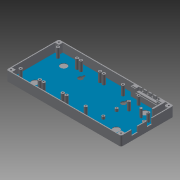
# Autodesk Inventor part: bottom-case
Saved by Autodesk Inventor 2015 (Build 190159000, 159)
## iProperties
Created: 2016-04-25
Part Number: bottom-case
Material: 一般
Document SubType Name: Modeling
Designer: yamashita1
Density: 1 g/cm^3
Appearance: 既定
Author: yamashita1
Autodesk Inventor part; units mm, degrees
ref_plane "YZ Plane" through (0, 0, 0) normal (1, 0, 0) x (0, 1, 0)
ref_plane "XZ Plane" through (0, 0, 0) normal (0, 1, 0) x (-1, 0, 0)
ref_plane "XY Plane" through (0, 0, 0) normal (0, 0, 1) x (1, 0, 0)
sketch "スケッチ1" plane through (0, 0, 0) normal (0, 0, 1) x (1, 0, 0)
  line L0 (-120, 55) -> (120, 55)
  line L1 (120, 55) -> (120, -55)
  line L2 (120, -55) -> (-120, -55)
  line L3 (-120, -55) -> (-120, 55)
  point P0 (0, 0)
  dimension "d0" = 240
  dimension "d1" = 110
  dimension "d2" = 120
  dimension "d3" = 55
  constraints: 8 end point, 2 parallel, 1 horizontal, 1 perpendicular
  measures "d0" distance of L1.end L2.end
  measures "d1" distance of L0.end L1.end
  measures "d2" distance from line of L3 point (0, 0)
  measures "d3" distance from line of L2 point (0, 0)
extrude "押し出し1" add sketch "スケッチ1" along normal blind 20
sketch "スケッチ2" plane through (0, 0, 20) normal (0, 0, 1) x (1, 0, 0)
  line L0 (-118, 53) -> (118, 53)
  line L1 (118, 53) -> (118, -53)
  line L2 (118, -53) -> (-118, -53)
  line L3 (-118, -53) -> (-118, 53)
  point P0 (0, 0)
  dimension "d6" = 236
  dimension "d7" = 106
  dimension "d8" = 118
  dimension "d9" = 53
  constraints: 8 end point, 2 parallel, 1 horizontal, 1 perpendicular
  measures "d6" distance of L1.end L2.end
  measures "d7" distance of L0.end L1.end
  measures "d8" distance from line of L3 point (0, 0)
  measures "d9" distance from line of L2 point (0, 0)
extrude "押し出し2" cut sketch "スケッチ2" against normal blind 18
sketch "スケッチ3" plane through (0, 0, 2) normal (0, 0, 1) x (1, 0, 0)
  line L0 (-118, 53) -> (-110, 53)
  line L1 (-110, 53) -> (-110, 45)
  line L2 (-110, 45) -> (-118, 45)
  line L3 (-118, 45) -> (-118, 53)
  line L4 (-118, -53) -> (-110, -53)
  line L5 (-110, -53) -> (-110, -45)
  line L6 (-110, -45) -> (-118, -45)
  line L7 (-118, -45) -> (-118, -53)
  line L8 (118, -53) -> (110, -53)
  line L9 (110, -53) -> (110, -45)
  line L10 (110, -45) -> (118, -45)
  line L11 (118, -45) -> (118, -53)
  line L12 (118, 53) -> (110, 53)
  line L13 (110, 53) -> (110, 45)
  line L14 (110, 45) -> (118, 45)
  line L15 (118, 45) -> (118, 53)
  point P0 (0, 0)
  dimension "d13" = 8
  dimension "d14" = 8
  dimension "d15" = 8
  dimension "d16" = 8
  dimension "d17" = 8
  dimension "d18" = 8
  dimension "d19" = 8
  dimension "d117" = 8
  constraints: 32 end point, 8 parallel, 4 horizontal, 4 perpendicular
  measures "d13" distance of L0.end L1.end
  measures "d14" distance of L6.end L5.end
  measures "d15" distance of L5.end L4.end
  measures "d16" distance of L9.end L10.end
  measures "d17" distance of L8.end L9.end
  measures "d18" distance of L14.end L13.end
  measures "d19" distance of L13.end L12.end
  measures "d117" distance from line of L3 L1.end
extrude "押し出し3" add sketch "スケッチ3" along normal blind 18
sketch "スケッチ4" plane through (0, 0, 20) normal (0, 0, 1) x (1, 0, 0)
  circle A0 centre (-115, 50) radius 1.6
  line L0 (-120, 55) -> (-120, -55) projected
  line L1 (120, 55) -> (-120, 55) projected
  circle A1 centre (-115, -50) radius 1.6
  line L2 (-120, -55) -> (120, -55) projected
  circle A2 centre (115, 50) radius 1.6
  line L3 (120, -55) -> (120, 55) projected
  circle A3 centre (115, -50) radius 1.6
  point P0 (0, 0)
  dimension "d22" = 3.2
  dimension "d23" = 5
  dimension "d24" = 5
  dimension "d25" = 3.2
  dimension "d26" = 5
  dimension "d27" = 5
  dimension "d28" = 3.2
  dimension "d29" = 5
  dimension "d30" = 5
  dimension "d31" = 3.2
  dimension "d32" = 5
  dimension "d33" = 5
  constraints: 4 centre point
  measures "d22" diameter of A0
  measures "d23" distance from line of L0 A0.centre
  measures "d24" distance from line of L1 A0.centre
  measures "d25" diameter of A1
  measures "d26" distance from line of L0 A1.centre
  measures "d27" distance from line of L2 A1.centre
  measures "d28" diameter of A2
  measures "d29" distance from line of L1 A2.centre
  measures "d30" distance from line of L3 A2.centre
  measures "d31" diameter of A3
  measures "d32" distance from line of L3 A3.centre
  measures "d33" distance from line of L2 A3.centre
extrude "押し出し4" cut sketch "スケッチ4" against normal blind 20 contours A0 | A1 | A2 | A3
sketch "スケッチ5" plane through (0, 0, 0) normal (0, 0, -1) x (-1, 0, 0)
  circle A0 centre (115, -50) radius 3.5
  circle A1 centre (115, -50) radius 1.6 projected
  circle A2 centre (115, 50) radius 3.5
  circle A3 centre (115, 50) radius 1.6 projected
  circle A4 centre (-115, 50) radius 3.5
  circle A5 centre (-115, 50) radius 1.6 projected
  circle A6 centre (-115, -50) radius 3.5
  circle A7 centre (-115, -50) radius 1.6 projected
  point P0 (0, 0)
  dimension "d36" = 7
  dimension "d37" = 7
  dimension "d38" = 7
  dimension "d39" = 7
  constraints: 4 centre point, 4 concentric
  measures "d36" diameter of A0
  measures "d37" diameter of A2
  measures "d38" diameter of A4
  measures "d39" diameter of A6
extrude "押し出し5" cut sketch "スケッチ5" against normal blind 15
sketch "スケッチ6" plane through (0, 0, 2) normal (0, 0, 1) x (1, 0, 0)
  circle A0 centre (-10, -39) radius 3.25
  circle A1 centre (-10, 39) radius 3.25
  circle A2 centre (30, 39) radius 3.25
  circle A3 centre (30, -39) radius 3.25
  point P0 (0, 0)
  dimension "d42" = 39
  dimension "d43" = 10
  dimension "d44" = 40
  dimension "d45" = 39
  dimension "d46" = 6.5
  dimension "d47" = 6.5
  dimension "d48" = 6.5
  dimension "d49" = 6.5
  constraints: 4 centre point, 4 coincident, 2 horizontal alignment, 2 vertical alignment
  measures "d42" vertical distance of point (-10, -39) point (0, 0)
  measures "d43" horizontal distance of point (-10, -39) point (0, 0)
  measures "d44" distance of point (30, -39) point (-10, -39)
  measures "d45" vertical distance of point (-10, 39) point (0, 0)
  measures "d46" diameter of A0
  measures "d47" diameter of A1
  measures "d48" diameter of A2
  measures "d49" diameter of A3
extrude "押し出し6" add sketch "スケッチ6" along normal blind 19.4
sketch "スケッチ7" plane through (-10, 39, 21.4) normal (0, 0, 1) x (1, 0, 0)
  circle A0 centre (0, 0) radius 1.4
  circle A1 centre (0, 0) radius 3.25 projected
  circle A2 centre (0, -78) radius 1.4
  circle A3 centre (0, -78) radius 3.25 projected
  circle A4 centre (40, 0) radius 1.4
  circle A5 centre (40, 0) radius 3.25 projected
  circle A6 centre (40, -78) radius 1.4
  circle A7 centre (40, -78) radius 3.25 projected
  point P0 (10, -39)
  dimension "d52" = 2.8
  dimension "d53" = 2.8
  dimension "d54" = 2.8
  dimension "d55" = 2.8
  constraints: 4 centre point, 4 concentric
  measures "d52" diameter of A0
  measures "d53" diameter of A2
  measures "d54" diameter of A4
  measures "d55" diameter of A6
extrude "押し出し7" cut sketch "スケッチ7" against normal blind 10 contours A0 | A2 | A4 | A6
pattern_linear "矩形状パターン1" count 3 spacing 48 along (-1, 0, 0) of "押し出し6", "押し出し7"
sketch "スケッチ8" plane through (120, -55, 0) normal (1, 0, 0) x (0, 0, -1)
  line L0 (-20, 100) -> (-20, 10) projected
  line L1 (-20, 21.9) -> (-9, 21.9)
  line L2 (-9, 21.9) -> (-9, 34.9)
  line L3 (-9, 34.9) -> (-20, 34.9)
  line L4 (-20, 34.9) -> (-20, 21.9)
  line L5 (-20, 0) -> (-20, 110) projected
  line L6 (-20, 54.515) -> (-9, 54.515)
  line L7 (-9, 54.515) -> (-9, 64.515)
  line L8 (-9, 64.515) -> (-20, 64.515)
  line L9 (-20, 64.515) -> (-20, 54.515)
  point P0 (0, 55)
  point P1 (-20, 66.5)
  point P2 (-20, 59.515)
  point P3 (-20, 28.4)
  dimension "d61" = 11.5
  dimension "d62" = 6.985
  dimension "d63" = 38.1
  dimension "d64" = 11
  dimension "d65" = 13
  dimension "d67" = 11
  dimension "d68" = 10
  dimension "d71" = 1.985
  dimension "d72" = 31.6
  constraints: 16 end point, 4 parallel, 3 point on line, 2 collinear, 2 horizontal, 2 perpendicular
  measures "d61" vertical distance of point (-20, 66.5) point (0, 55)
  measures "d62" distance of point (-20, 59.515) point (-20, 66.5)
  measures "d63" distance of point (-20, 28.4) point (-20, 66.5)
  measures "d64" distance of L3.end L2.end
  measures "d65" distance of L2.end L1.end
  measures "d67" distance of L8.end L7.end
  measures "d68" distance of L7.end L6.end
  measures "d71" vertical distance of L7.end point (-20, 66.5)
  measures "d72" vertical distance of L2.end point (-20, 66.5)
extrude "押し出し8" cut sketch "スケッチ8" against normal blind 2
sketch "スケッチ9" plane through (0, 0, 2) normal (0, 0, 1) x (1, 0, 0)
  line L0 (118, 45) -> (118, 9.515) projected
  circle A0 centre (104.03, 8.96) radius 3
  circle A1 centre (51.96, 3.88) radius 3
  circle A2 centre (51.96, -24.06) radius 3
  circle A3 centre (102.76, -39.3) radius 3
  point P0 (0, 0)
  point P1 (118, 11.5)
  dimension "d75" = 11.5
  dimension "d76" = 13.97
  dimension "d77" = 2.54
  dimension "d78" = 66.04
  dimension "d79" = 7.62
  dimension "d80" = 27.94
  dimension "d81" = 15.24
  dimension "d82" = 50.8
  dimension "d83" = 6
  constraints: 4 centre point, 4 coincident, 3 equal radius, 1 point on line, 1 vertical alignment
  measures "d75" vertical distance of point (118, 11.5) point (0, 0)
  measures "d76" horizontal distance of point (104.03, 8.96) point (118, 11.5)
  measures "d77" vertical distance of point (104.03, 8.96) point (118, 11.5)
  measures "d78" horizontal distance of point (51.96, 3.88) point (118, 11.5)
  measures "d79" vertical distance of point (51.96, 3.88) point (118, 11.5)
  measures "d80" distance of point (51.96, -24.06) point (51.96, 3.88)
  measures "d81" horizontal distance of point (102.76, -39.3) point (118, 11.5)
  measures "d82" vertical distance of point (102.76, -39.3) point (118, 11.5)
  measures "d83" diameter of A0
extrude "押し出し9" add sketch "スケッチ9" along normal blind 5.2
sketch "スケッチ10" plane through (104.03, 8.96, 7.2) normal (0, 0, 1) x (1, 0, 0)
  circle A0 centre (0, 0) radius 1.4
  circle A1 centre (0, 0) radius 3 projected
  circle A2 centre (-52.07, -5.08) radius 1.4
  circle A3 centre (-52.07, -33.02) radius 1.4
  circle A4 centre (-52.07, -5.08) radius 3 projected
  circle A5 centre (-52.07, -33.02) radius 3 projected
  point P0 (-104.03, -8.96)
  dimension "d86" = 2.8
  constraints: 3 centre point, 3 concentric, 2 equal radius
  measures "d86" diameter of A0
extrude "押し出し10" cut sketch "スケッチ10" against normal blind 5.2 contours A0 | A2 | A3
sketch "スケッチ11" plane through (-120, 55, 0) normal (0, 1, 0) x (1, 0, 0)
  line L0 (230, -20) -> (10, -20) projected
  line L1 (209.24, -20) -> (205.24, -20)
  line L2 (205.24, -20) -> (205.24, -14.5)
  line L3 (205.24, -14.5) -> (209.24, -14.5)
  line L4 (209.24, -14.5) -> (209.24, -20)
  line L5 (240, -20) -> (0, -20) projected
  point P0 (120, 0)
  point P1 (192, -20)
  point P2 (207.24, -20)
  point P3 (207.24, -14.5)
  dimension "d89" = 72
  dimension "d90" = 15.24
  dimension "d91" = 4
  dimension "d92" = 5.5
  constraints: 8 end point, 2 parallel, 2 point on line, 1 collinear, 1 horizontal, 1 midpoint, 1 perpendicular, 1 vertical alignment
  measures "d89" horizontal distance of point (192, -20) point (120, 0)
  measures "d90" distance of point (207.24, -20) point (192, -20)
  measures "d91" distance of L2.end L3.end
  measures "d92" distance of L1.end L2.end
extrude "押し出し11" cut sketch "スケッチ11" against normal blind 2
pattern_linear "矩形状パターン2" count 4 spacing 10.16 along (-1, 0, 0) of "押し出し11"
sketch "スケッチ12" plane through (0, 0, 2) normal (0, 0, 1) x (1, 0, 0)
  line L0 (-110, 53) -> (110, 53) projected
  line L1 (40, 53) -> (104, 53)
  line L2 (104, 53) -> (104, 45)
  line L3 (104, 45) -> (40, 45)
  line L4 (40, 45) -> (40, 53)
  line L5 (68.92, 53) -> (75.08, 53) projected
  line L6 (89.24, 53) -> (110, 53) projected
  point P0 (0, 0)
  point P1 (72, 53)
  point P2 (72, 45)
  point P3 (72, 53)
  dimension "d98" = 72
  dimension "d99" = 64
  dimension "d100" = 8
  constraints: 8 end point, 2 midpoint, 2 parallel, 1 collinear, 1 horizontal, 1 perpendicular, 1 point on line, 1 vertical alignment
  measures "d98" horizontal distance of point (72, 53) point (0, 0)
  measures "d99" distance of L2.end L3.end
  measures "d100" distance of L1.end L2.end
extrude "押し出し12" add sketch "スケッチ12" along normal blind 18
sketch "スケッチ13" plane through (0, 0, 20) normal (0, 0, 1) x (1, 0, 0)
  line L0 (75.08, 55) -> (68.92, 55) projected
  line L1 (42, 48) -> (102, 48)
  line L2 (102, 48) -> (102, 46.2)
  line L3 (102, 46.2) -> (42, 46.2)
  line L4 (42, 46.2) -> (42, 48)
  point P0 (0, 0)
  point P1 (72, 55)
  point P2 (72, 46.2)
  point P3 (72, 55)
  dimension "d103" = 60
  dimension "d104" = 1.8
  dimension "d105" = 7
  constraints: 8 end point, 3 midpoint, 2 parallel, 1 horizontal, 1 perpendicular, 1 vertical alignment
  measures "d103" distance of L2.end L3.end
  measures "d104" distance of L1.end L2.end
  measures "d105" vertical distance of L1.start point (72, 55)
extrude "押し出し13" cut sketch "スケッチ13" against normal blind 11
sketch "スケッチ14" plane through (0, 0, 20) normal (0, 0, 1) x (1, 0, 0)
  line L0 (75.08, 55) -> (68.92, 55) projected
  line L1 (49.5, 53) -> (94.5, 53)
  line L2 (94.5, 53) -> (94.5, 48)
  line L3 (94.5, 48) -> (49.5, 48)
  line L4 (49.5, 48) -> (49.5, 53)
  point P0 (0, 0)
  point P1 (72, 55)
  point P2 (72, 48)
  point P3 (72, 55)
  dimension "d108" = 45
  dimension "d109" = 5
  dimension "d110" = 2
  constraints: 8 end point, 3 midpoint, 2 parallel, 1 horizontal, 1 perpendicular, 1 vertical alignment
  measures "d108" distance of L2.end L3.end
  measures "d109" distance of L1.end L2.end
  measures "d110" vertical distance of L1.start point (72, 55)
extrude "押し出し14" cut sketch "スケッチ14" against normal blind 6.8
sketch "スケッチ15" plane through (0, 0, 20) normal (0, 0, 1) x (1, 0, 0)
  line L0 (75.08, 55) -> (68.92, 55) projected
  line L1 (49.5, 45) -> (94.5, 45)
  line L2 (94.5, 45) -> (94.5, 47.5)
  line L3 (94.5, 47.5) -> (49.5, 47.5)
  line L4 (49.5, 47.5) -> (49.5, 45)
  line L5 (40, 45) -> (104, 45) projected
  point P0 (0, 0)
  point P1 (72, 55)
  point P2 (72, 45)
  point P3 (72, 55)
  dimension "d113" = 45
  dimension "d114" = 2.5
  constraints: 8 end point, 3 midpoint, 2 parallel, 1 collinear, 1 horizontal, 1 perpendicular, 1 vertical alignment
  measures "d113" distance of L3.end L2.end
  measures "d114" distance of L2.end L1.end
extrude "押し出し15" cut sketch "スケッチ15" against normal blind 7.5
sketch "スケッチ16" plane through (0, 0, 2) normal (0, 0, 1) x (1, 0, 0)
  circle A0 centre (104.32, 38.16) radius 3
  circle A1 centre (63.68, 38.16) radius 3
  circle A2 centre (63.68, 17.84) radius 3
  circle A3 centre (104.32, 17.84) radius 3
  circle A4 centre (89.08, 17.84) radius 2.5
  point P0 (0, 0)
  point P1 (84, 28)
  dimension "d118" = 84
  dimension "d119" = 28
  dimension "d120" = 20.32
  dimension "d121" = 10.16
  dimension "d122" = 20.32
  dimension "d123" = 10.16
  dimension "d124" = 6
  dimension "d125" = 5.08
  dimension "d126" = 5
  constraints: 5 centre point, 5 coincident, 3 equal radius, 3 horizontal alignment, 2 vertical alignment
  measures "d118" horizontal distance of point (84, 28) point (0, 0)
  measures "d119" vertical distance of point (0, 0) point (84, 28)
  measures "d120" horizontal distance of point (104.32, 38.16) point (84, 28)
  measures "d121" vertical distance of point (84, 28) point (104.32, 38.16)
  measures "d122" horizontal distance of point (84, 28) point (63.68, 38.16)
  measures "d123" vertical distance of point (104.32, 17.84) point (84, 28)
  measures "d124" diameter of A0
  measures "d125" horizontal distance of point (84, 28) point (89.08, 17.84)
  measures "d126" diameter of A4
extrude "押し出し16" add sketch "スケッチ16" along normal blind 16.7
sketch "スケッチ17" plane through (104.32, 38.16, 18.7) normal (0, 0, 1) x (1, 0, 0)
  circle A0 centre (0, 0) radius 1.4
  circle A1 centre (-40.64, 0) radius 1.4
  circle A2 centre (-40.64, -20.32) radius 1.4
  circle A3 centre (0, -20.32) radius 1.4
  circle A4 centre (0, 0) radius 3 projected
  circle A5 centre (-40.64, 0) radius 3 projected
  circle A6 centre (-40.64, -20.32) radius 3 projected
  circle A7 centre (0, -20.32) radius 3 projected
  point P0 (-104.32, -38.16)
  dimension "d129" = 2.8
  constraints: 4 centre point, 4 concentric, 3 equal radius
  measures "d129" diameter of A0
extrude "押し出し17" cut sketch "スケッチ17" against normal blind 10 contours A0 | A1 | A2 | A3
sketch "スケッチ18" plane through (0, 0, 2) normal (0, 0, 1) x (1, 0, 0)
  line L0 (113.5, 40.5) -> (116.5, 40.5)
  line L1 (116.5, 40.5) -> (116.5, 15.5)
  line L2 (116.5, 15.5) -> (113.5, 15.5)
  line L3 (113.5, 15.5) -> (113.5, 40.5)
  point P0 (0, 0)
  point P1 (84, 28)
  point P2 (115, 28)
  point P3 (116.5, 28)
  point P4 (115, 15.5)
  dimension "d132" = 84
  dimension "d133" = 28
  dimension "d134" = 31
  dimension "d135" = 3
  dimension "d136" = 25
  constraints: 8 end point, 2 horizontal alignment, 2 midpoint, 2 parallel, 1 horizontal, 1 perpendicular, 1 vertical alignment
  measures "d132" horizontal distance of point (84, 28) point (0, 0)
  measures "d133" vertical distance of point (84, 28) point (0, 0)
  measures "d134" distance of point (115, 28) point (84, 28)
  measures "d135" distance of L1.end L2.end
  measures "d136" distance of L0.end L1.end
extrude "押し出し18" add sketch "スケッチ18" along normal blind 29.5
fillet "フィレット1" radius 3 4 edges at (120, -55, 10) (120, 55, 10) (-120, -55, 10) (-120, 55, 10)
sketch "スケッチ19" plane through (0, 0, 2) normal (0, 0, 1) x (1, 0, 0)
  circle A0 centre (-45, 25) radius 5
  circle A1 centre (45, 25) radius 5
  circle A2 centre (-45, 33) radius 2
  circle A3 centre (45, 33) radius 2
  line L0 (-47, 33) -> (-43, 33)
  line L1 (-43, 33) -> (-43, 29)
  line L2 (-43, 29) -> (-47, 29)
  line L3 (-47, 29) -> (-47, 33)
  line L4 (43, 33) -> (47, 33)
  line L5 (47, 33) -> (47, 29)
  line L6 (47, 29) -> (43, 29)
  line L7 (43, 29) -> (43, 33)
  point P0 (0, 0)
  dimension "d146" = 4
  dimension "d147" = 4
  dimension "d140" = 25
  dimension "d141" = 45
  dimension "d142" = 45
  dimension "d143" = 10
  dimension "d144" = 10
  dimension "d145" = 8
  dimension "d148" = 4
  dimension "d149" = 4
  dimension "d150" = 4
  dimension "d151" = 4
  constraints: 16 end point, 6 coincident, 4 horizontal alignment, 4 parallel, 2 centre point, 2 horizontal, 2 midpoint, 2 perpendicular, 2 vertical alignment, 4 other
  measures "d140" vertical distance of point (-45, 25) point (0, 0)
  measures "d141" horizontal distance of point (-45, 25) point (0, 0)
  measures "d142" horizontal distance of point (45, 25) point (0, 0)
  measures "d143" diameter of A0
  measures "d144" diameter of A1
  measures "d145" distance of point (-45, 33) A0.centre
  measures "d148" distance of L1.end L2.end
  measures "d149" distance of L0.end L1.end
  measures "d150" distance of L5.end L6.end
  measures "d151" distance of L4.end L5.end
extrude "押し出し19" cut sketch "スケッチ19" against normal blind 2
sketch "スケッチ20" plane through (0, 0, 2) normal (0, 0, 1) x (1, 0, 0)
  circle A0 centre (85, 30) radius 7
  circle A1 centre (-85, 30) radius 7
  circle A2 centre (-85, -30) radius 7
  circle A3 centre (85, -30) radius 7
  point P0 (0, 0)
  dimension "d154" = 30
  dimension "d155" = 85
  dimension "d156" = 85
  dimension "d157" = 30
  dimension "d158" = 14
  constraints: 4 centre point, 4 coincident, 3 equal radius, 2 horizontal alignment, 2 vertical alignment
  measures "d154" vertical distance of point (85, 30) point (0, 0)
  measures "d155" horizontal distance of point (85, 30) point (0, 0)
  measures "d156" horizontal distance of point (-85, 30) point (0, 0)
  measures "d157" vertical distance of point (85, -30) point (0, 0)
  measures "d158" diameter of A0
extrude "押し出し20" cut sketch "スケッチ20" against normal blind 1
equation "\"d2\" = 0.5 * d0"
equation "\"d3\" = 0.5 * d1"
equation "\"d8\" = 0.5 * d6"
equation "\"d9\" = 0.5 * d7"
equation "\"d45\" = d42"
equation "\"d71\" = d62 - 0.5 * d68"
equation "\"d72\" = d63 - 0.5 * d65"
equation "\"d122\" = d120"
equation "\"d123\" = d121"
equation "\"d142\" = d141"
equation "\"d156\" = d155"
equation "\"d157\" = d154"
